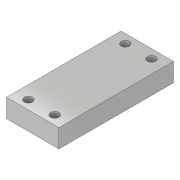
# Autodesk Inventor part: MotorMountSpacer
Saved by Autodesk Inventor 2017.3 (Build 213256000, 256)
## iProperties
Created: 2017-06-08
Part Number: MotorMountSpacer
Material: Aluminum 6061
Document SubType Name: Modeling
Designer: Michael
Density: 2.7 g/cm^3
Appearance: Aluminum - Dark
Author: Michael
Autodesk Inventor part; units mm, degrees
ref_plane "YZ Plane" through (0, 0, 0) normal (1, 0, 0) x (0, 1, 0)
ref_plane "XZ Plane" through (0, 0, 0) normal (0, 1, 0) x (-1, 0, 0)
ref_plane "XY Plane" through (0, 0, 0) normal (0, 0, 1) x (1, 0, 0)
sketch "Sketch1" plane through (0, 0, 0) normal (0, 1, 0) x (-1, 0, 0)
  line L0 (9.02, 19.685) -> (-9.02, 19.685)
  line L1 (-9.02, 19.685) -> (-9.02, -19.685)
  line L2 (-9.02, -19.685) -> (9.02, -19.685)
  line L3 (9.02, -19.685) -> (9.02, 19.685)
  circle A0 centre (4.51, 16.6309) radius 1.4224
  circle A1 centre (-4.51, 16.6309) radius 1.4224
  circle A2 centre (4.51, -16.6309) radius 1.4224
  circle A3 centre (-4.51, -16.6309) radius 1.4224
  point P0 (0, 0)
  dimension "d0" = 39.37
  dimension "d1" = 19.685
  dimension "d2" = 18.04
  dimension "d3" = 9.02
  dimension "d4" = 4.51
  dimension "d5" = 3.0541
  dimension "d6" = 2.8448
  dimension "d7" = 3.0541
  dimension "d8" = 3.0541
  dimension "d9" = 3.0541
  dimension "d10" = 2.8448
  dimension "d11" = 2.8448
  dimension "d12" = 2.8448
  dimension "d13" = 4.51
  dimension "d14" = 4.51
  dimension "d15" = 4.51
  constraints: 8 end point, 4 centre point, 2 parallel, 1 horizontal, 1 perpendicular
  measures "d0" distance of L0.end L1.end
  measures "d1" distance from line of L0 point (0, 0)
  measures "d2" distance between parallel lines of L1 L3
  measures "d3" distance from line of L3 point (0, 0)
  measures "d4" distance from line of L3 A0.centre
  measures "d5" distance from line of L0 A0.centre
  measures "d6" diameter of A0
  measures "d7" distance from line of L0 A1.centre
  measures "d8" distance from line of L2 A2.centre
  measures "d9" distance from line of L2 A3.centre
  measures "d10" diameter of A1
  measures "d11" diameter of A3
  measures "d12" diameter of A2
  measures "d13" distance from line of L1 A1.centre
  measures "d14" distance from line of L1 A3.centre
  measures "d15" distance from line of L3 A2.centre
extrude "Extrusion1" add sketch "Sketch1" along normal blind 6.35
equation "\"d1\" = 0.5 * d0"
equation "\"d3\" = 0.5 * d2"
equation "\"d7\" = d5"
equation "\"d8\" = d5"
equation "\"d9\" = d5"
equation "\"d10\" = d6"
equation "\"d11\" = d10"
equation "\"d12\" = d6"
equation "\"d13\" = d4"
equation "\"d14\" = d4"
equation "\"d15\" = d4"
body "Solid1"
